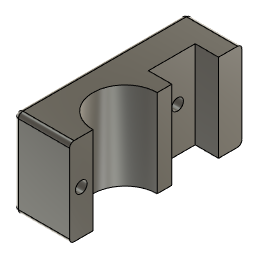
ConectorEstruturaGK_16 (Autodesk Fusion 360 design; units mm, degrees)
Autodesk Fusion 360 part; units mm, degrees
sketch "Esboço1" plane through (0, 0, 0) normal (0, 0, 1) x (1, 0, 0)
  line L0 (1.9999, 62) -> (21, 62)
  line L1 (21, 62) -> (21, 54)
  line L2 (21, 54) -> (13, 54)
  line L3 (13, 54) -> (13, 38)
  line L4 (13, 38) -> (21, 38)
  arc A0 (21, 33) -> (21, 11) centre (21, 22) ccw
  line L5 (21, 11) -> (21, 3)
  line L6 (2, 3) -> (2, 62)
  line L7 (2, 3) -> (21, 3)
  line L8 (21, 33) -> (21, 38)
  line L9 (1.9999, 62) -> (2, 62)
  dimension "d1" = 11
  dimension "d2" = 16
  dimension "d3" = 8
  dimension "d5" = 8
  dimension "d8" = 8
  dimension "d10" = 8
  dimension "d35" = 5
  dimension "d36" = 19
  constraint perpendicular L1 L2
  constraint perpendicular L2 L3
  constraint perpendicular L3 L4
  constraint vertical L5
  constraint perpendicular L5 L7
  measures "d1" distance of A0.end A0.centre
  measures "d2" distance of L2.end L3.end
  measures "d3" distance of L1.end L2.end
  measures "d5" distance of L0.end L1.end
  measures "d8" distance of L4.end L3.end
  measures "d10" distance of A0.end L5.end
  measures "d35" distance of L4.end A0.start
  measures "d36" distance of L0.end L6.end
extrude "Extrusão1" add sketch "Esboço1" along normal blind 30
hole "Furo2" at (2, 7, 15) direction (1, 0, 0) diameter 4 depth 21 tip angle 180
hole "Furo3" at (2, 48, 15) direction (1, 0, 0) diameter 4 depth 21 tip angle 180
fillet "Arredondamento4" radius 1.5 8 edges at (11.5, 62, 30) (2, 62, 15) (2, 32.5, 30) (2, 32.5, 0) (2, 3, 15) (11.5, 3, 0) (11.5, 3, 30) (11.5, 62, 0)
